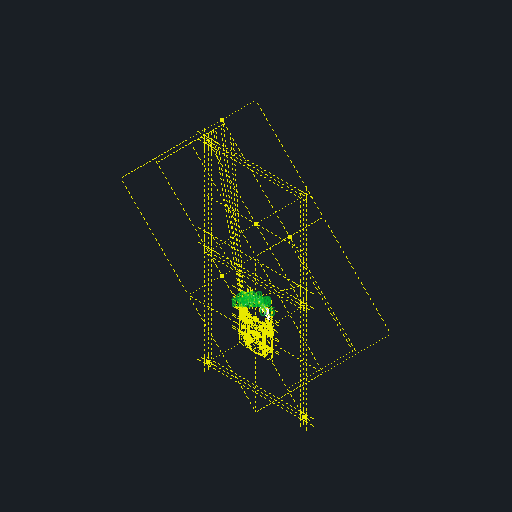
# Autodesk Inventor part: sensorcircuit
Saved by Autodesk Inventor 2023.5 (Build 275446000, 446)
## iProperties
Created: 2025-01-11
Part Number: sensorcircuit
Material: 一般
Document SubType Name: Modeling
Designer: IshiiLabHonda
Density: 1 g/cm^3
Appearance: 既定
Author: IshiiLabHonda
Autodesk Inventor part; units mm, degrees
ref_plane "YZ Plane" through (0, 0, 0) normal (1, 0, 0) x (0, 1, 0)
ref_plane "XZ Plane" through (0, 0, 0) normal (0, 1, 0) x (-1, 0, 0)
ref_plane "XY Plane" through (0, 0, 0) normal (0, 0, 1) x (1, 0, 0)
derived "circuit.ipt"
sketch "スケッチ1" plane through (0, 0, 0) normal (0, 0, 1) x (1, 0, 0)
  line L0 (0, 0) -> (0, 1) construction
  line L1 (0, 0) -> (1, 0) construction
  line L2 (-90, 90) -> (90, 90) construction
  line L3 (90, 90) -> (90, -90) construction
  line L4 (90, -90) -> (-90, -90) construction
  line L5 (-90, -90) -> (-90, 90) construction
  line L6 (-90, -90) -> (90, 90) construction
  line L7 (-90, 90) -> (90, -90) construction
  line L8 (-84, 96) -> (-84, 84) construction
  line L9 (-84, 84) -> (-96, 84) construction
  line L10 (-96, 84) -> (-96, 96) construction
  line L11 (-96, 96) -> (-84, 84) construction
  line L12 (-84, 96) -> (-96, 84) construction
  line L13 (-96, 96) -> (-84, 96) construction
  line L14 (-96, -96) -> (-96, -84) construction
  line L15 (-84, -96) -> (-96, -96) construction
  line L16 (-96, -96) -> (-84, -84) construction
  line L17 (-96, -84) -> (-84, -96) construction
  line L18 (-84, -84) -> (-84, -96) construction
  line L19 (-96, -84) -> (-84, -84) construction
  line L20 (96, -96) -> (84, -96) construction
  line L21 (96, -84) -> (96, -96) construction
  line L22 (96, -96) -> (84, -84) construction
  line L23 (84, -96) -> (96, -84) construction
  line L24 (84, -84) -> (96, -84) construction
  line L25 (84, -96) -> (84, -84) construction
  line L26 (96, 96) -> (96, 84) construction
  line L27 (84, 96) -> (96, 96) construction
  line L28 (96, 96) -> (84, 84) construction
  line L29 (96, 84) -> (84, 96) construction
  line L30 (84, 84) -> (84, 96) construction
  line L31 (96, 84) -> (84, 84) construction
  line L32 (-84, 84) -> (-84, -84) construction
  line L33 (-96, 84) -> (-96, -84) construction
  line L34 (-84, -84) -> (84, -84) construction
  line L35 (-84, -96) -> (84, -96) construction
  line L36 (96, 84) -> (96, -84) construction
  line L37 (84, 84) -> (84, -84) construction
  line L38 (-84, 96) -> (84, 96) construction
  line L39 (-84, 84) -> (84, 84) construction
  line L40 (-19, 15) -> (19, 15) construction
  line L41 (19, 15) -> (19, -15) construction
  line L42 (19, -15) -> (-19, -15) construction
  line L43 (-19, -15) -> (-19, 15) construction
  line L44 (-19, 15) -> (19, -15) construction
  line L45 (19, 15) -> (-19, -15) construction
  line L46 (-30.25, 11.5) -> (-19, 11.5) construction
  line L47 (-19, -11.5) -> (-30.25, -11.5) construction
  line L48 (-30.25, -11.5) -> (-30.25, 11.5) construction
  line L49 (-30.25, 11.5) -> (-19, -11.5) construction
  line L50 (-19, 11.5) -> (-30.25, -11.5) construction
  line L51 (30.25, 11.5) -> (19, 11.5) construction
  line L52 (19, -11.5) -> (30.25, -11.5) construction
  line L53 (30.25, -11.5) -> (30.25, 11.5) construction
  line L54 (30.25, 11.5) -> (19, -11.5) construction
  line L55 (19, 11.5) -> (30.25, -11.5) construction
  line L56 (-19, -10) -> (19, -10) construction
  line L57 (-19, -12.5) -> (19, -12.5) construction
  line L58 (-19, 10) -> (19, 10) construction
  line L59 (-19, 12.5) -> (19, 12.5) construction
  line L60 (-16.5, -15) -> (-16.5, 15) construction
  line L61 (16.5, -15) -> (16.5, 15) construction
  line L62 (-12.5, -10) -> (-12.5, -15) construction
  line L63 (-16.5, -10) -> (-12.5, -15) construction
  line L64 (-16.5, -15) -> (-12.5, -10) construction
  circle A0 centre (-14.5, -12.5) radius 0.8 construction
  line L65 (12.5, -10) -> (12.5, -15) construction
  line L66 (16.5, -10) -> (12.5, -15) construction
  line L67 (16.5, -15) -> (12.5, -10) construction
  circle A1 centre (14.5, -12.5) radius 0.8 construction
  line L68 (-12.5, 10) -> (-12.5, 15) construction
  line L69 (-16.5, 10) -> (-12.5, 15) construction
  line L70 (-16.5, 15) -> (-12.5, 10) construction
  circle A2 centre (-14.5, 12.5) radius 0.8 construction
  line L71 (12.5, 10) -> (12.5, 15) construction
  line L72 (16.5, 10) -> (12.5, 15) construction
  circle A3 centre (14.5, 12.5) radius 0.8 construction
  line L73 (16.5, 15) -> (12.5, 10) construction
  line L74 (-96, 276) -> (-84, 276) construction
  line L75 (-84, 276) -> (-84, 264) construction
  line L76 (-84, 264) -> (-96, 264) construction
  line L77 (-96, 264) -> (-96, 276) construction
  line L78 (-96, 276) -> (-84, 264) construction
  line L79 (-84, 276) -> (-96, 264) construction
  line L80 (-90, 90) -> (-90, 270) construction
  line L81 (-96, 264) -> (-96, 96) construction
  line L82 (-84, 264) -> (-84, 96) construction
  line L83 (96, 276) -> (84, 276) construction
  line L84 (84, 276) -> (84, 264) construction
  line L85 (84, 264) -> (96, 264) construction
  line L86 (96, 264) -> (96, 276) construction
  line L87 (96, 276) -> (84, 264) construction
  line L88 (84, 276) -> (96, 264) construction
  line L89 (90, 90) -> (90, 270) construction
  line L90 (96, 264) -> (96, 96) construction
  line L91 (84, 264) -> (84, 96) construction
  line L92 (-84, 276) -> (84, 276) construction
  line L93 (-84, 264) -> (84, 264) construction
  line L94 (-90, 270) -> (90, 270) construction
  line L95 (-90, 270) -> (90, 90) construction
  line L96 (-90, 90) -> (90, 270) construction
  circle A4 centre (0, 0) radius 15 construction
  line L97 (-96, 120) -> (96, 120) construction
  line L98 (0, 127.2792) -> (0, -127.2792) construction
  line L99 (-127.2792, 0) -> (127.2792, 0) construction
  line L100 (127.2792, 0) -> (0, -127.2792) construction
  line L101 (0, -127.2792) -> (-127.2792, 0) construction
  line L102 (-127.2792, 0) -> (0, 127.2792) construction
  line L103 (0, 127.2792) -> (127.2792, 0) construction
  line L104 (127.2792, 254.5584) -> (254.5584, 127.2792) construction
  line L105 (254.5584, 127.2792) -> (127.2792, 0) construction
  line L106 (127.2792, 0) -> (0, 127.2792) construction
  line L107 (0, 127.2792) -> (127.2792, 254.5584) construction
  line L108 (-127.2792, 254.5584) -> (0, 127.2792) construction
  line L109 (0, 127.2792) -> (-127.2792, 0) construction
  line L110 (-127.2792, 0) -> (-254.5584, 127.2792) construction
  line L111 (-254.5584, 127.2792) -> (-127.2792, 254.5584) construction
  line L112 (0, 381.8377) -> (127.2792, 254.5584) construction
  line L113 (127.2792, 254.5584) -> (0, 127.2792) construction
  line L114 (0, 127.2792) -> (-127.2792, 254.5584) construction
  line L115 (-127.2792, 254.5584) -> (0, 381.8377) construction
  line L116 (190.9188, 63.6396) -> (63.6396, 190.9188) construction
  line L117 (-190.9188, 190.9188) -> (-63.6396, 63.6396) construction
  line L118 (59.397, -59.397) -> (186.6762, 67.8823) construction
  line L119 (59.397, 186.6762) -> (186.6762, 59.397) construction
  line L120 (63.6396, 190.9188) -> (-63.6396, 318.1981) construction
  line L121 (-186.6762, 186.6762) -> (-59.397, 313.9554) construction
  point P0 (-90, -90)
  point P1 (90, -90)
  point P2 (-24.625, 0)
  point P3 (-84, 120)
  point P4 (84, 120)
  point P5 (0, 0)
sketch "スケッチ5" plane through (0, 0, 0) normal (0, 0, 1) x (1, 0, 0)
  line L0 (0, 0) -> (0, 1) construction
  line L1 (30.25, 11.5) -> (19, 11.5) construction
  line L2 (19, 11.5) -> (30.25, -11.5) construction
  line L3 (30.25, 11.5) -> (19, -11.5) construction
  line L4 (30.25, -11.5) -> (30.25, 11.5) construction
  line L5 (19, -11.5) -> (30.25, -11.5) construction
  line L6 (-90, 90) -> (90, 90) construction
  line L7 (-90, -90) -> (90, 90) construction
  line L8 (-90, 90) -> (90, -90) construction
  line L9 (-84, 84) -> (-84, -84) construction
  line L10 (-96, 84) -> (-96, -84) construction
  line L11 (-90, -90) -> (-90, 90) construction
  line L12 (-84, 84) -> (-96, 84) construction
  line L13 (-96, 84) -> (-96, 96) construction
  line L14 (84, 84) -> (84, -84) construction
  line L15 (90, 90) -> (90, -90) construction
  line L16 (96, 84) -> (84, 84) construction
  line L17 (96, 84) -> (96, -84) construction
  line L18 (90, -90) -> (-90, -90) construction
  line L19 (-84, -84) -> (84, -84) construction
  line L20 (-84, -96) -> (84, -96) construction
  line L21 (-84, -84) -> (-84, -96) construction
  line L22 (-96, -96) -> (-96, -84) construction
  line L23 (-84, -96) -> (-96, -96) construction
  line L24 (-96, -96) -> (-84, -84) construction
  line L25 (-96, -84) -> (-84, -96) construction
  line L26 (-96, -84) -> (-84, -84) construction
  line L27 (0, 0) -> (1, 0) construction
  line L28 (-84, 264) -> (-96, 264) construction
  line L29 (-96, 276) -> (-84, 276) construction
  line L30 (-96, 264) -> (-96, 276) construction
  line L31 (-84, 276) -> (-96, 264) construction
  line L32 (-96, 276) -> (-84, 264) construction
  line L33 (-84, 276) -> (-84, 264) construction
  line L34 (84, -96) -> (84, -84) construction
  line L35 (96, -96) -> (84, -96) construction
  line L36 (96, -84) -> (96, -96) construction
  line L37 (96, -96) -> (84, -84) construction
  line L38 (84, -96) -> (96, -84) construction
  line L39 (84, -84) -> (96, -84) construction
  line L40 (-19, 15) -> (19, 15) construction
  line L41 (19, 15) -> (19, -15) construction
  line L42 (16.5, 15) -> (12.5, 10) construction
  line L43 (12.5, 10) -> (12.5, 15) construction
  line L44 (16.5, 10) -> (12.5, 15) construction
  line L45 (16.5, -15) -> (16.5, 15) construction
  line L46 (-19, 10) -> (19, 10) construction
  line L47 (-19, 12.5) -> (19, 12.5) construction
  circle A0 centre (0, 0) radius 15 construction
  line L48 (-19, -10) -> (19, -10) construction
  line L49 (-19, -12.5) -> (19, -12.5) construction
  line L50 (19, -15) -> (-19, -15) construction
  line L51 (-19, 15) -> (19, -15) construction
  line L52 (19, 15) -> (-19, -15) construction
  line L53 (-16.5, -15) -> (-16.5, 15) construction
  line L54 (-19, -15) -> (-19, 15) construction
  line L55 (-30.25, 11.5) -> (-19, 11.5) construction
  line L56 (-19, -11.5) -> (-30.25, -11.5) construction
  line L57 (-30.25, -11.5) -> (-30.25, 11.5) construction
  line L58 (-30.25, 11.5) -> (-19, -11.5) construction
  line L59 (-19, 11.5) -> (-30.25, -11.5) construction
  line L60 (-12.5, 10) -> (-12.5, 15) construction
  circle A1 centre (-14.5, 12.5) radius 0.8 construction
  line L61 (-16.5, 10) -> (-12.5, 15) construction
  line L62 (-16.5, 15) -> (-12.5, 10) construction
  circle A2 centre (14.5, 12.5) radius 0.8 construction
  line L63 (-84, 96) -> (-96, 84) construction
  line L64 (-96, 96) -> (-84, 96) construction
  line L65 (-84, 96) -> (-84, 84) construction
  line L66 (-96, 96) -> (-84, 84) construction
  line L67 (-96, 264) -> (-96, 96) construction
  line L68 (-84, 264) -> (-84, 96) construction
  line L69 (-84, 96) -> (84, 96) construction
  line L70 (-84, 84) -> (84, 84) construction
  line L71 (84, 84) -> (84, 96) construction
  line L72 (96, 96) -> (96, 84) construction
  line L73 (96, 96) -> (84, 84) construction
  line L74 (96, 84) -> (84, 96) construction
  line L75 (-96, 120) -> (96, 120) construction
  line L76 (84, 96) -> (96, 96) construction
  line L77 (-84, 264) -> (84, 264) construction
  line L78 (84, 264) -> (84, 96) construction
  line L79 (-84, 276) -> (84, 276) construction
  line L80 (96, 264) -> (96, 96) construction
  line L81 (-90, 270) -> (90, 270) construction
  line L82 (-90, 270) -> (90, 90) construction
  line L83 (-90, 90) -> (90, 270) construction
  line L84 (90, 90) -> (90, 270) construction
  line L85 (-90, 90) -> (-90, 270) construction
  line L86 (84, 264) -> (96, 264) construction
  line L87 (96, 276) -> (84, 276) construction
  line L88 (96, 276) -> (84, 264) construction
  line L89 (84, 276) -> (96, 264) construction
  line L90 (96, 264) -> (96, 276) construction
  line L91 (84, 276) -> (84, 264) construction
  circle A3 centre (-14.5, -12.5) radius 0.8 construction
  line L92 (-12.5, -10) -> (-12.5, -15) construction
  line L93 (-16.5, -15) -> (-12.5, -10) construction
  line L94 (12.5, -10) -> (12.5, -15) construction
  circle A4 centre (14.5, -12.5) radius 0.8 construction
  line L95 (16.5, -15) -> (12.5, -10) construction
  line L96 (16.5, -10) -> (12.5, -15) construction
  line L97 (-16.5, -10) -> (-12.5, -15) construction
  line L98 (-12.9773, 53.9269) -> (-10.5199, 55.6476) construction
  line L99 (-8.7991, 53.1902) -> (-12.9773, 53.9269) construction
  circle A5 centre (-10.8882, 53.5585) radius 0.8 construction
  line L100 (-8.7991, 53.1902) -> (-11.2566, 51.4694) projected
  line L101 (-10.5199, 55.6476) -> (-11.2566, 51.4694) construction
  line L102 (-11.2566, 51.4694) -> (-12.9773, 53.9269) projected
  line L103 (-30.25, 44.8844) -> (-31, 44.3592) construction
  line L104 (-12.9471, 57) -> (-30.25, 44.8844) construction
  line L105 (-30.25, 57) -> (-31, 57) construction
  line L106 (-10.5199, 55.6476) -> (-8.7991, 53.1902) projected
  line L107 (-30.25, 57) -> (30.25, 57) construction
  line L108 (-6.2185, 52.5556) -> (-11.543, 48.8274) projected
  line L109 (-11.543, 48.8274) -> (-15.558, 54.5615) projected
  line L110 (-10.2335, 58.2897) -> (-6.2185, 52.5556) projected
  line L111 (1.0005, 57) -> (-30.25, 35.1182) construction
  line L112 (-1.0005, 57) -> (30.25, 35.1182) construction
  line L113 (-19, 15) -> (19, 15) construction
  line L114 (12.5, 10) -> (12.5, 15) construction
  line L115 (-19, 10) -> (19, 10) construction
  circle A6 centre (-14.5, 12.5) radius 0.8 construction
  line L116 (-12.5, 10) -> (-12.5, 15) construction
  line L117 (-16.5, 10) -> (-12.5, 15) construction
  line L118 (-16.5, 15) -> (-12.5, 10) construction
  line L119 (-19, 12.5) -> (19, 12.5) construction
  line L120 (30.25, 57) -> (31, 57) construction
  line L121 (30.25, 11.5) -> (30.25, 57) construction
  line L122 (-6.1403, 52) -> (6.1403, 52) construction
  line L123 (-30.25, 35.1182) -> (-31, 34.593) construction
  line L124 (-30.25, 11.5) -> (-30.25, 57) construction
  line L125 (-6.7921, 53.3748) -> (-12.1165, 49.6465) construction
  line L126 (-10.8882, 53.5585) -> (-10.4294, 52.9032) construction
  line L127 (-10.8882, 53.5585) -> (-10.2329, 54.0174) construction
  line L128 (-6.2185, 52.5556) -> (-15.558, 54.5615) construction
  line L129 (-9.6599, 57.4705) -> (-14.9844, 53.7423) construction
  line L130 (-15.558, 54.5615) -> (-10.2335, 58.2897) construction
  line L131 (-10.2335, 58.2897) -> (-11.543, 48.8274) construction
  line L132 (-30.25, 11.5) -> (-19, 11.5) construction
  line L133 (-30.25, 11.5) -> (-19, -11.5) construction
  line L134 (30.25, 11.5) -> (19, 11.5) construction
  line L135 (30.25, -11.5) -> (30.25, 11.5) construction
  line L136 (19, 11.5) -> (30.25, -11.5) construction
  line L137 (30.25, 11.5) -> (19, -11.5) construction
  line L138 (0, 0) -> (0, 1) construction
  line L139 (0, 0) -> (1, 0) construction
  circle A7 centre (0, 0) radius 7.5 construction
  circle A8 centre (0, 0) radius 15 construction
  line L140 (-16.5, -15) -> (-16.5, 15) construction
  circle A9 centre (14.5, 12.5) radius 0.8 construction
  line L141 (-12.5, -10) -> (-12.5, -15) construction
  line L142 (12.5, -10) -> (12.5, -15) construction
  line L143 (16.5, 10) -> (12.5, 15) construction
  line L144 (-16.5, -15) -> (-12.5, -10) construction
  line L145 (16.5, -10) -> (12.5, -15) construction
  line L146 (16.5, 15) -> (12.5, 10) construction
  line L147 (-19, -12.5) -> (19, -12.5) construction
  line L148 (19, -15) -> (-19, -15) construction
  line L149 (-19, 11.5) -> (-30.25, -11.5) construction
  line L150 (19, -11.5) -> (30.25, -11.5) construction
  line L151 (-19, -11.5) -> (-30.25, -11.5) construction
  line L152 (-30.25, -11.5) -> (-30.25, 11.5) construction
  line L153 (16.5, -15) -> (16.5, 15) construction
  line L154 (19, 15) -> (19, -15) construction
  line L155 (-19, -15) -> (-19, 15) construction
  line L156 (-19, 15) -> (19, -15) construction
  line L157 (19, 15) -> (-19, -15) construction
  line L158 (-31, -8.5) -> (31, -8.5) construction
  line L159 (-31, 8.5) -> (31, 8.5) construction
  line L160 (-31, -30) -> (31, -30) construction
  line L161 (-31, 57) -> (-31, -30) construction
  line L162 (31, 57) -> (31, -30) construction
  line L163 (84, -84) -> (96, -84) construction
  line L164 (84, -96) -> (96, -84) construction
  line L165 (96, -96) -> (84, -84) construction
  line L166 (96, -84) -> (96, -96) construction
  line L167 (96, -96) -> (84, -96) construction
  line L168 (-96, 84) -> (-96, -84) construction
  line L169 (-84, 84) -> (-84, -84) construction
  line L170 (-90, -90) -> (-90, 90) construction
  line L171 (-84, -84) -> (84, -84) construction
  line L172 (-84, -96) -> (84, -96) construction
  line L173 (-90, -90) -> (90, 90) construction
  line L174 (90, -90) -> (-90, -90) construction
  line L175 (-90, 90) -> (90, -90) construction
  line L176 (84, 84) -> (84, -84) construction
  line L177 (90, 90) -> (90, -90) construction
  line L178 (96, 84) -> (96, -84) construction
  line L179 (84, -96) -> (84, -84) construction
  line L180 (-19, -10) -> (19, -10) construction
  circle A10 centre (14.5, -12.5) radius 0.8 construction
  line L181 (16.5, -15) -> (12.5, -10) construction
  line L182 (-16.5, -10) -> (-12.5, -15) construction
  line L183 (-84, -84) -> (-84, -96) construction
  line L184 (-96, -84) -> (-84, -84) construction
  line L185 (-84, -96) -> (-96, -96) construction
  line L186 (-96, -96) -> (-84, -84) construction
  line L187 (-96, -84) -> (-84, -96) construction
  line L188 (-96, -96) -> (-96, -84) construction
  circle A11 centre (-14.5, -12.5) radius 0.8 construction
  line L189 (-96, 96) -> (-84, 96) construction
  line L190 (-84, 96) -> (-84, 84) construction
  line L191 (-84, 96) -> (-96, 84) construction
  line L192 (-96, 96) -> (-84, 84) construction
  line L193 (84, 96) -> (96, 96) construction
  line L194 (96, 84) -> (84, 84) construction
  line L195 (96, 96) -> (96, 84) construction
  line L196 (96, 96) -> (84, 84) construction
  line L197 (96, 84) -> (84, 96) construction
  line L198 (-96, 120) -> (96, 120) construction
  line L199 (-84, 96) -> (84, 96) construction
  line L200 (-90, 90) -> (90, 90) construction
  line L201 (-84, 84) -> (-96, 84) construction
  line L202 (-96, 84) -> (-96, 96) construction
  line L203 (-84, 84) -> (84, 84) construction
  line L204 (84, 120) -> (-30.25, 40.0013) construction
  line L205 (-84, 120) -> (30.25, 40.0013) construction
  line L206 (84, 84) -> (84, 96) construction
  line L207 (-84, 264) -> (-96, 264) construction
  line L208 (-90, 90) -> (-90, 270) construction
  line L209 (-96, 264) -> (-96, 96) construction
  line L210 (-84, 264) -> (-84, 96) construction
  line L211 (96, 264) -> (96, 96) construction
  line L212 (84, 264) -> (84, 96) construction
  line L213 (90, 90) -> (90, 270) construction
  line L214 (-90, 90) -> (90, 270) construction
  line L215 (-90, 270) -> (90, 90) construction
  line L216 (-84, 264) -> (84, 264) construction
  line L217 (-90, 270) -> (90, 270) construction
  line L218 (-96, 264) -> (-96, 276) construction
  line L219 (-96, 276) -> (-84, 276) construction
  line L220 (-96, 276) -> (-84, 264) construction
  line L221 (-84, 276) -> (-96, 264) construction
  line L222 (-84, 276) -> (-84, 264) construction
  line L223 (-84, 276) -> (84, 276) construction
  line L224 (84, 264) -> (96, 264) construction
  line L225 (96, 264) -> (96, 276) construction
  line L226 (96, 276) -> (84, 264) construction
  line L227 (96, 276) -> (84, 276) construction
  line L228 (84, 276) -> (96, 264) construction
  line L229 (84, 276) -> (84, 264) construction
  line L230 (-31, 8.5) -> (-19, 8.5) construction
  line L231 (-31, -8.5) -> (-19, -8.5) construction
  line L232 (-19, 8.5) -> (-19, -8.5) construction
  circle A12 centre (0, 0) radius 7.5 construction
  line L233 (31, 8.5) -> (19, 8.5) construction
  line L234 (31, -8.5) -> (19, -8.5) construction
  line L235 (19, 8.5) -> (19, -8.5) construction
  line L236 (31, 8.5) -> (31, 8.5) projected
  line L237 (-31, -8.5) -> (-12.9594, -30) construction
  line L238 (-12.9594, -30) -> (12.9594, -30) construction
  line L239 (31, -8.5) -> (12.9594, -30) construction
  circle A13 centre (-14.5, 12.5) radius 1 construction
  circle A14 centre (14.5, 12.5) radius 1 construction
  circle A15 centre (-14.5, -12.5) radius 1 construction
  circle A16 centre (14.5, -12.5) radius 1 construction
  line L240 (-10.5199, 55.6476) -> (-12.9773, 53.9269) projected
  line L241 (-12.9773, 53.9269) -> (-11.2566, 51.4694) construction
  line L242 (-11.2566, 51.4694) -> (-8.7991, 53.1902) construction
  line L243 (-8.7991, 53.1902) -> (-10.5199, 55.6476) construction
  line L244 (-26.25, 26.5) -> (-26.3613, 27.2922) construction
  line L245 (-26.25, 26.5) -> (-25.4578, 26.6113) construction
  circle A17 centre (-26.25, 26.5) radius 0.8 construction
  line L246 (-24.1223, 29.3236) -> (-23.4264, 24.3723) construction
  line L247 (-28.3777, 23.6764) -> (-29.0736, 28.6277) construction
  line L248 (-24.1223, 29.3236) -> (-28.3777, 23.6764) construction
  line L249 (-29.0736, 28.6277) -> (-24.1223, 29.3236) construction
  line L250 (-23.4264, 24.3723) -> (-28.3777, 23.6764) construction
  line L251 (-29.0736, 28.6277) -> (-23.4264, 24.3723) construction
  line L252 (10.5199, 55.6476) -> (12.9773, 53.9269) projected
  line L253 (12.9773, 53.9269) -> (11.2566, 51.4694) projected
  line L254 (11.2566, 51.4694) -> (8.7991, 53.1902) projected
  line L255 (8.7991, 53.1902) -> (10.5199, 55.6476) projected
  line L256 (-29.0736, 28.6277) -> (-28.3777, 23.6764) construction
  line L257 (-24.1223, 29.3236) -> (-19.1709, 30.0195) construction
  line L258 (-19.1709, 30.0195) -> (-18.4751, 25.0681) construction
  line L259 (-18.4751, 25.0681) -> (-23.4264, 24.3723) construction
  line L260 (28.3777, 23.6764) -> (23.4264, 24.3723) construction
  line L261 (18.4751, 25.0681) -> (23.4264, 24.3723) construction
  line L262 (19.1709, 30.0195) -> (18.4751, 25.0681) construction
  line L263 (24.1223, 29.3236) -> (19.1709, 30.0195) construction
  line L264 (24.1223, 29.3236) -> (29.0736, 28.6277) construction
  line L265 (29.0736, 28.6277) -> (28.3777, 23.6764) construction
  line L266 (-29.0736, 28.6277) -> (-19.1709, 30.0195) construction
  line L267 (-18.4751, 25.0681) -> (-19.1709, 30.0195) projected
  line L268 (-18.4751, 25.0681) -> (-28.3777, 23.6764) construction
  line L269 (19.1709, 30.0195) -> (29.0736, 28.6277) construction
  line L270 (28.3777, 23.6764) -> (29.0736, 28.6277) construction
  line L271 (28.3777, 23.6764) -> (18.4751, 25.0681) construction
  line L272 (19.1709, 30.0195) -> (18.4751, 25.0681) construction
  line L273 (-9.6771, 59.2897) -> (9.6771, 59.2897) construction
  line L274 (-9.6771, 59.2897) -> (-9.6771, 59.2897) construction
  line L275 (-3.6771, 59.2897) -> (-0.9296, 58.2897) construction
  line L276 (-0.9296, 58.2897) -> (0.9296, 58.2897) construction
  line L277 (0.9296, 58.2897) -> (3.6771, 59.2897) construction
  line L278 (-4.6137, 54.2897) -> (4.6137, 54.2897) construction
  line L279 (-18.1736, 44.795) -> (-4.6137, 54.2897) construction
  line L280 (-31, 8.5) -> (-22.0451, 50.6295) construction
  line L281 (-22.0451, 50.6295) -> (-9.6771, 59.2897) construction
  line L282 (31, 8.5) -> (22.0451, 50.6295) construction
  line L283 (-18.1736, 44.795) -> (-23.6565, 19) construction
  line L284 (18.1736, 44.795) -> (23.6565, 19) construction
  line L285 (-23.6565, 19) -> (23.6565, 19) construction
  line L286 (-17.5234, -20) -> (17.5234, -20) construction
  line L287 (17.5234, -20) -> (12.3689, -25) construction
  line L288 (12.3689, -25) -> (-12.3689, -25) construction
  line L289 (-12.3689, -25) -> (-17.5234, -20) construction
  line L290 (-31, -8.5) -> (-31, -12.5) construction
  line L291 (-31, -12.5) -> (-12.9594, -30) construction
  line L292 (31, -8.5) -> (31, -12.5) construction
  line L293 (31, -12.5) -> (12.9594, -30) construction
  line L294 (-31, 8.5) -> (-31, 26.5) construction
  line L295 (-31, 26.5) -> (-26.3435, 30.4073) construction
  line L296 (31, 8.5) -> (31, 26.5) construction
  line L297 (31, 26.5) -> (26.3435, 30.4073) construction
  line L298 (-8.9594, -30) -> (-7.4594, -28.5) construction
  line L299 (-7.4594, -28.5) -> (7.4594, -28.5) construction
  line L300 (7.4594, -28.5) -> (8.9594, -30) construction
  line L301 (18.1736, 44.795) -> (4.6137, 54.2897) construction
  line L302 (22.0451, 50.6295) -> (9.6771, 59.2897) construction
  line L303 (-23.6565, 19) -> (-24.8255, 13.5) construction
  line L304 (-24.8255, 13.5) -> (-20.8255, 13.5) construction
  line L305 (-20.8255, 13.5) -> (-15.3255, 19) construction
  line L306 (23.6565, 19) -> (24.8255, 13.5) construction
  line L307 (24.8255, 13.5) -> (20.8255, 13.5) construction
  line L308 (20.8255, 13.5) -> (15.3255, 19) construction
  line L309 (-17.5234, -20) -> (-24.2242, -13.5) construction
  line L310 (-24.2242, -13.5) -> (-21.2242, -13.5) construction
  line L311 (-21.2242, -13.5) -> (-11.5234, -20) construction
  line L312 (17.5234, -20) -> (24.2242, -13.5) construction
  line L313 (24.2242, -13.5) -> (21.2242, -13.5) construction
  line L314 (21.2242, -13.5) -> (11.5234, -20) construction
  line L315 (-10.5173, 23.5) -> (-4.5173, 23.5) projected
  line L316 (-4.5173, 23.5) -> (-2, 26.5) projected
  line L317 (-2, 26.5) -> (2, 26.5) projected
  line L318 (2, 26.5) -> (4.5173, 23.5) projected
  line L319 (4.5173, 23.5) -> (10.5173, 23.5) projected
  line L320 (0, 0) -> (1, 0) construction
  line L321 (0, 0) -> (0, 1) construction
  line L322 (-30.5, 13) -> (-20, 13) projected
  line L323 (-20, 13) -> (-20, 17.5) projected
  line L324 (-20, 17.5) -> (-16, 17.5) projected
  line L325 (20, 17.5) -> (16, 17.5) projected
  line L326 (20, 13) -> (20, 17.5) projected
  line L327 (30.5, 13) -> (20, 13) projected
  circle A18 centre (0, 0) radius 1.5 projected
  line L328 (-16, 17.5) -> (-16, -17) projected
  line L329 (16, 17.5) -> (16, -17) projected
  line L330 (-30.5, 20.6916) -> (-10.5173, 23.5) projected
  line L331 (30.5, 20.6916) -> (10.5173, 23.5) projected
  circle A19 centre (-10.0234, -17) radius 0.475 construction
  circle A20 centre (-10.0234, -17) radius 0.8 projected
  circle A21 centre (-10.0234, -17) radius 1.5 projected
  line L332 (-11.5234, -20) -> (-11.5234, -15) construction
  circle A22 centre (10.0234, -17) radius 0.475 construction
  circle A23 centre (10.0234, -17) radius 0.8 projected
  circle A24 centre (10.0234, -17) radius 1.5 projected
  circle A25 centre (-9, 15.5) radius 0.475 construction
  circle A26 centre (-9, 15.5) radius 0.8 projected
  circle A27 centre (-9, 15.5) radius 1.5 projected
  circle A28 centre (9, 15.5) radius 0.475 construction
  circle A29 centre (9, 15.5) radius 0.8 projected
  circle A30 centre (9, 15.5) radius 1.5 projected
  line L333 (-9.091, 59.0897) -> (-21.597, 50.3329)
  line L334 (-21.597, 50.3329) -> (-23.6677, 40.5908)
  line L335 (-3.4267, 53.2897) -> (3.4267, 53.2897)
  line L336 (23.5225, 41.2738) -> (21.597, 50.3329)
  line L337 (21.597, 50.3329) -> (9.091, 59.0897)
  line L338 (9.091, 59.0897) -> (-9.091, 59.0897)
  circle A31 centre (-17.3746, 49.0168) radius 0.475 construction
  circle A32 centre (-17.3746, 49.0168) radius 0.8 projected
  circle A33 centre (-17.3746, 49.0168) radius 1.5 construction
  circle A34 centre (17.3746, 49.0168) radius 0.475 construction
  circle A35 centre (17.3746, 49.0168) radius 0.8 projected
  circle A36 centre (17.3746, 49.0168) radius 1.5 construction
  line L339 (-11.6471, 47.5337) -> (-10.6006, 47.0457)
  line L340 (-10.6006, 47.0457) -> (-4.8665, 51.0607)
  line L341 (-4.8665, 51.0607) -> (-4.9672, 52.211)
  line L342 (-16.3711, 44.2259) -> (-11.6471, 47.5337)
  line L343 (-4.9672, 52.211) -> (-3.4267, 53.2897)
  line L344 (11.6471, 47.5337) -> (10.6006, 47.0457)
  line L345 (10.6006, 47.0457) -> (4.8665, 51.0607)
  line L346 (4.8665, 51.0607) -> (4.9672, 52.211)
  line L347 (4.9672, 52.211) -> (3.4267, 53.2897)
  line L348 (0, 59.0897) -> (-10.3891, 58.1808)
  line L349 (0, 59.0897) -> (10.3891, 58.1808)
  line L350 (-10.3891, 58.1808) -> (-2.3891, 58.1808)
  line L351 (-2.3891, 58.1808) -> (0, 59.0897)
  line L352 (10.3891, 58.1808) -> (2.3891, 58.1808)
  line L353 (2.3891, 58.1808) -> (0, 59.0897)
  line L354 (-3.1638, 53.2897) -> (-1, 51.4741)
  line L355 (-1, 51.4741) -> (1, 51.4741)
  line L356 (1, 51.4741) -> (3.1638, 53.2897)
  line L357 (-10, -29) -> (10, -29) projected
  line L358 (-16, -17) -> (-22.863, -17) projected
  line L359 (-22.863, -17) -> (-22.863, -19) projected
  line L360 (16, -17) -> (22.863, -17) projected
  line L361 (22.863, -17) -> (22.863, -19) projected
  line L362 (-12.8008, -25) -> (-18.1572, -23.5648) projected
  line L363 (-18.1572, -23.5648) -> (-22.863, -19) projected
  line L364 (12.8008, -25) -> (18.1572, -23.5648) projected
  line L365 (18.1572, -23.5648) -> (22.863, -19) projected
  line L366 (-30.5, 13) -> (-30.5, 20.6916) projected
  line L367 (30.5, 13) -> (30.5, 20.6916) projected
  line L368 (-16.3711, 44.2259) -> (-16.2403, 42.7317)
  line L369 (-16.2403, 42.7317) -> (-24.4318, 36.9959)
  line L370 (-24.4318, 36.9959) -> (-23.6677, 40.5908)
  line L371 (16.3711, 44.2259) -> (16.2403, 42.7317)
  line L372 (16.2403, 42.7317) -> (24.4318, 36.9959)
  line L373 (11.6471, 47.5337) -> (16.3711, 44.2259)
  line L374 (23.5225, 41.2738) -> (24.4318, 36.9959)
  line L375 (-12.8008, -25) -> (-10, -29) projected
  line L376 (10, -29) -> (12.8008, -25) projected
  line L377 (-1.25, 25) -> (1.25, 25) projected
  line L378 (2, 24.25) -> (2, 24.25) projected
  line L379 (1.25, 23.5) -> (-1.25, 23.5) projected
  line L380 (-2, 24.25) -> (-2, 24.25) projected
  arc A37 (-1.25, 25) -> (-2, 24.25) centre (-1.25, 24.25) ccw projected
  arc A38 (-2, 24.25) -> (-1.25, 23.5) centre (-1.25, 24.25) ccw projected
  arc A39 (1.25, 23.5) -> (2, 24.25) centre (1.25, 24.25) ccw projected
  arc A40 (2, 24.25) -> (1.25, 25) centre (1.25, 24.25) ccw projected
  line L381 (-30.5, 20.6916) -> (-28.3474, 27.0531) projected
  line L382 (-28.3474, 27.0531) -> (-19.435, 28.3057) projected
  line L383 (-19.435, 28.3057) -> (-15.6123, 22.7839) projected
  line L384 (30.5, 20.6916) -> (28.3474, 27.0531) projected
  line L385 (28.3474, 27.0531) -> (19.435, 28.3057) projected
  line L386 (19.435, 28.3057) -> (15.6123, 22.7839) projected
  line L387 (-30.8721, 30.6471) -> (-17.9987, 32.4563) projected
  line L388 (-17.9987, 32.4563) -> (-16.6765, 23.0488) projected
  line L389 (-16.6765, 23.0488) -> (-29.55, 21.2395) projected
  line L390 (-29.55, 21.2395) -> (-30.8721, 30.6471) projected
  line L391 (-22.0451, 50.6295) -> (-18.1736, 44.795) construction
  line L392 (-21.8107, 27.6837) -> (-26, 24.1685) construction
  line L393 (-26, 24.1685) -> (-26, 13.5) construction
  line L394 (-24.8255, 13.5) -> (-26, 13.5) construction
  line L395 (21.8107, 27.6837) -> (26, 24.1685) projected
  line L396 (26, 24.1685) -> (26, 13.5) projected
  line L397 (24.8255, 13.5) -> (26, 13.5) projected
  circle A41 centre (-28.5, 18.5) radius 0.475 construction
  circle A42 centre (-28.5, 18.5) radius 0.8 projected
  circle A43 centre (-28.5, 18.5) radius 1.5 projected
  line L398 (-19.435, 28.3057) -> (-10.5173, 23.5) projected
  line L399 (19.435, 28.3057) -> (10.5173, 23.5) projected
  circle A44 centre (28.5, 18.5) radius 0.8 projected
  circle A45 centre (28.5, 18.5) radius 1.5 projected
  circle A46 centre (28.5, 18.5) radius 0.475 construction
  line L400 (-12.9471, 57) -> (12.9471, 57) projected
  line L401 (10.2335, 58.2897) -> (6.2185, 52.5556) projected
  line L402 (6.2185, 52.5556) -> (11.543, 48.8274) projected
  line L403 (11.543, 48.8274) -> (15.558, 54.5615) projected
  circle A47 centre (-6.875, 0) radius 0.9 projected
  circle A48 centre (-6.875, 0) radius 0.8 construction
  circle A49 centre (6.875, 0) radius 0.8 construction
  circle A50 centre (6.875, 0) radius 0.9 projected
  circle A51 centre (0, 0) radius 5.75 projected
  circle A52 centre (-6.875, 0) radius 0.625 construction
  circle A53 centre (0, 0) radius 4.25 projected
  line L404 (30.8721, 30.6471) -> (17.9987, 32.4563) projected
  line L405 (17.9987, 32.4563) -> (16.6765, 23.0488) projected
  line L406 (16.6765, 23.0488) -> (29.55, 21.2395) projected
  line L407 (29.55, 21.2395) -> (30.8721, 30.6471) projected
  point P0 (-90, -90)
  point P1 (90, -90)
  point P2 (-24.625, 0)
  point P3 (-8.226, 55.4227)
  point P4 (-5.9733, 57)
  point P5 (0, 61.1826)
  point P6 (-24.625, 0)
  point P7 (-90, -90)
  point P8 (90, -90)
  point P9 (-5.9733, 57)
  point P10 (5.9733, 57)
  point P11 (10.3891, 58.1808)
  point P12 (10.3891, 58.1808)
  point P13 (-2, 25)
  point P14 (-2, 23.5)
  point P15 (0.6109, 58.1808)
  point P16 (-0.6109, 58.1808)
  point P17 (0.6109, 58.1808)
  point P18 (10.1572, 58.1808)
  point P19 (-10.1572, 58.1808)
  dimension "d2" = 0.5
  dimension "d3" = 0.5
  dimension "d5" = 0.5
  dimension "d13" = 1
  dimension "d14" = 0.5
  dimension "d15" = 120
  dimension "d16" = 120
  dimension "d17" = 0.5
  dimension "d18" = 1.5
  dimension "d19" = 7
  dimension "d21" = 0.2
  dimension "d22" = 5
  dimension "d26" = 8
  dimension "d29" = 40
  dimension "d34" = 2
  dimension "d35" = 6.3276
  dimension "d39" = 120
  dimension "d40" = 10
  dimension "d41" = 1.5
  constraints: 62 end point, 13 horizontal alignment, 11 parallel, 3 point on line, 1 coincident, 1 collinear, 1 horizontal, 1 midpoint, 1 symmetric about line, 34 other
  measures "d2" distance between parallel lines of L333 L104
  measures "d3" distance between parallel lines of L280 L334
  measures "d5" distance between parallel lines of L282 L336
  measures "d13" distance between parallel lines of L335 L278
  measures "d14" distance between parallel lines of L343 L111
  measures "d15" angle of L341 L343
  measures "d16" angle of L342 L339
  measures "d17" distance between parallel lines of L342 L111
  measures "d18" distance between parallel lines of L340 L111
  measures "d19" distance of L339.end L340.end
  measures "d21" distance between parallel lines of L338 L273
  measures "d22" angle of L348 L338
  measures "d26" distance of L348.end L350.end
  measures "d29" angle of L354 L335
  measures "d34" distance of L354.end L355.end
  measures "d35" distance of L356.end L354.start
  measures "d39" angle of L368 L342
  measures "d40" distance of L368.end L369.end
  measures "d41" distance of L342.start L368.end
extrude "押し出し4" add sketch "スケッチ5" against normal blind 0.6 contours L110 L400 L401 L402 L403 L337 L336 L374 L372 L371 L373 L344 L345 L346 L347 L335 L343 L341 L340 L339 L342 L368 L369 L370 L334 L333 L109 L108 | L108 L109 L333 L400 L110 | L400 L333 L350 L110 | L110 L350 L351 L353 L352 L401 L400 | L350 L348 L110 | L110 L348 L351 L350 | L401 L352 L337 L400 | L400 L337 L403 L402 L401 | L348 L333 L110 | L110 L333 L338 L348 | L401 L349 L352 | L352 L353 L349 L401 | L338 L337 L401 L349 | L349 L401 L337
extrude "押し出し5" cut sketch "スケッチ5" against normal blind 0.6 contours L350 L348 L110 | L110 L348 L351 L350 | L401 L349 L352 | L352 L353 L349 L401
extrude "押し出し6" add sketch "スケッチ5" against normal blind 0.6 contours L335 L356 L355 L354
extrude "押し出し8" cut sketch "スケッチ5" against normal blind 0.6 contours L348 L333 L110 | L110 L333 L338 L348 | L338 L337 L401 L349 | L349 L401 L337
extrude "押し出し9" add sketch "スケッチ5" against normal blind 0.6 contours L350 L348 L110 | L110 L348 L351 L350 | L401 L349 L352 | L352 L353 L349 L401
extrude "押し出し10" cut sketch "スケッチ5" against normal blind 0.6 contours L350 L348 L110 | L110 L348 L351 L350 | L401 L349 L352 | L352 L353 L349 L401
extrude "押し出し11" cut sketch "スケッチ5" against normal blind 0.1 contours L401 L352 L337 L400 | L400 L337 L403 L402 L401
extrude "押し出し12" cut sketch "スケッチ5" against normal blind 0.1 contours L108 L109 L333 L400 L110 | L400 L333 L350 L110
sketch "スケッチ4" plane through (0, 0, 0) normal (0, 0, 1) x (1, 0, 0)
  line L0 (-84, 264) -> (-96, 264) construction
  line L1 (-90, 90) -> (-90, 270) construction
  line L2 (-96, 264) -> (-96, 96) construction
  line L3 (-96, 96) -> (-84, 96) construction
  line L4 (-84, 96) -> (-84, 84) construction
  line L5 (-84, 96) -> (-96, 84) construction
  line L6 (-96, 96) -> (-84, 84) construction
  line L7 (-84, 264) -> (-84, 96) construction
  line L8 (-84, 84) -> (-96, 84) construction
  line L9 (84, -84) -> (96, -84) construction
  line L10 (84, -96) -> (96, -84) construction
  line L11 (96, -96) -> (84, -84) construction
  line L12 (96, -84) -> (96, -96) construction
  line L13 (96, -96) -> (84, -96) construction
  line L14 (0, 0) -> (0, 1) construction
  line L15 (0, 0) -> (1, 0) construction
  line L16 (16.5, 15) -> (12.5, 10) construction
  line L17 (-96, 84) -> (-96, -84) construction
  line L18 (-84, 84) -> (-84, -84) construction
  line L19 (-90, -90) -> (-90, 90) construction
  line L20 (-90, 90) -> (90, 90) construction
  line L21 (-84, -84) -> (84, -84) construction
  line L22 (-84, -96) -> (84, -96) construction
  line L23 (-90, -90) -> (90, 90) construction
  line L24 (90, -90) -> (-90, -90) construction
  line L25 (-90, 90) -> (90, -90) construction
  line L26 (84, 84) -> (84, -84) construction
  line L27 (90, 90) -> (90, -90) construction
  line L28 (96, 84) -> (96, -84) construction
  line L29 (-96, 84) -> (-96, 96) construction
  line L30 (-84, -84) -> (-84, -96) construction
  line L31 (-96, -84) -> (-84, -84) construction
  line L32 (-84, -96) -> (-96, -96) construction
  line L33 (-96, -96) -> (-84, -84) construction
  line L34 (-96, -84) -> (-84, -96) construction
  line L35 (-96, -96) -> (-96, -84) construction
  line L36 (84, -96) -> (84, -84) construction
  line L37 (-19, -15) -> (-19, 15) construction
  line L38 (-30.25, 11.5) -> (-19, 11.5) construction
  line L39 (-19, -11.5) -> (-30.25, -11.5) construction
  line L40 (-19, 11.5) -> (-30.25, -11.5) construction
  line L41 (-30.25, 11.5) -> (-19, -11.5) construction
  line L42 (-30.25, -11.5) -> (-30.25, 11.5) construction
  line L43 (12.5, 10) -> (12.5, 15) construction
  circle A0 centre (14.5, 12.5) radius 0.8 construction
  line L44 (30.25, 11.5) -> (19, 11.5) construction
  line L45 (16.5, 10) -> (12.5, 15) construction
  circle A1 centre (14.5, -12.5) radius 0.8 construction
  line L46 (16.5, -15) -> (12.5, -10) construction
  line L47 (16.5, -10) -> (12.5, -15) construction
  line L48 (12.5, -10) -> (12.5, -15) construction
  circle A2 centre (-14.5, -12.5) radius 0.8 construction
  line L49 (-12.5, -10) -> (-12.5, -15) construction
  line L50 (-16.5, -15) -> (-12.5, -10) construction
  line L51 (-16.5, -10) -> (-12.5, -15) construction
  line L52 (96, 84) -> (84, 84) construction
  line L53 (96, 96) -> (96, 84) construction
  line L54 (84, 96) -> (96, 96) construction
  line L55 (96, 96) -> (84, 84) construction
  line L56 (84, 84) -> (84, 96) construction
  line L57 (96, 84) -> (84, 96) construction
  line L58 (-96, 264) -> (-96, 276) construction
  line L59 (-84, 276) -> (-84, 264) construction
  line L60 (-96, 276) -> (-84, 276) construction
  line L61 (-96, 276) -> (-84, 264) construction
  line L62 (-84, 276) -> (-96, 264) construction
  line L63 (-84, 84) -> (84, 84) construction
  line L64 (-84, 96) -> (84, 96) construction
  line L65 (84, 264) -> (84, 96) construction
  line L66 (90, 90) -> (90, 270) construction
  line L67 (-90, 90) -> (90, 270) construction
  line L68 (-90, 270) -> (90, 90) construction
  line L69 (96, 264) -> (96, 96) construction
  line L70 (-96, 120) -> (96, 120) construction
  line L71 (-84, 264) -> (84, 264) construction
  line L72 (-84, 276) -> (84, 276) construction
  line L73 (-90, 270) -> (90, 270) construction
  line L74 (84, 276) -> (84, 264) construction
  line L75 (84, 264) -> (96, 264) construction
  line L76 (96, 264) -> (96, 276) construction
  line L77 (96, 276) -> (84, 264) construction
  line L78 (96, 276) -> (84, 276) construction
  line L79 (84, 276) -> (96, 264) construction
  line L80 (-19, 15) -> (19, 15) construction
  line L81 (19, 15) -> (19, -15) construction
  line L82 (19, -15) -> (-19, -15) construction
  circle A3 centre (-14.5, 12.5) radius 0.8 construction
  line L83 (-16.5, 10) -> (-12.5, 15) construction
  line L84 (-12.5, 10) -> (-12.5, 15) construction
  line L85 (-16.5, 15) -> (-12.5, 10) construction
  circle A4 centre (0, 0) radius 15 construction
  line L86 (-19, 10) -> (19, 10) construction
  line L87 (-19, 12.5) -> (19, 12.5) construction
  line L88 (-19, 15) -> (19, -15) construction
  line L89 (19, 15) -> (-19, -15) construction
  line L90 (-19, -10) -> (19, -10) construction
  line L91 (-19, -12.5) -> (19, -12.5) construction
  line L92 (16.5, -15) -> (16.5, 15) construction
  line L93 (19, 11.5) -> (30.25, -11.5) construction
  line L94 (19, -11.5) -> (30.25, -11.5) construction
  line L95 (30.25, -11.5) -> (30.25, 11.5) construction
  line L96 (30.25, 11.5) -> (19, -11.5) construction
  line L97 (-16.5, -15) -> (-16.5, 15) construction
  line L98 (-84, 120) -> (30.25, 40.0013) construction
  line L99 (84, 120) -> (-30.25, 40.0013) construction
  line L100 (-30.25, 57) -> (30.25, 57) construction
  line L101 (1.0005, 57) -> (-30.25, 35.1182) construction
  line L102 (-1.0005, 57) -> (30.25, 35.1182) construction
  line L103 (-12.9471, 57) -> (-30.25, 44.8844) construction
  line L104 (-10.2335, 58.2897) -> (-6.2185, 52.5556) construction
  line L105 (-6.2185, 52.5556) -> (-11.543, 48.8274) construction
  line L106 (-11.543, 48.8274) -> (-15.558, 54.5615) construction
  line L107 (-15.558, 54.5615) -> (-10.2335, 58.2897) construction
  line L108 (-10.2335, 58.2897) -> (-11.543, 48.8274) construction
  line L109 (-6.2185, 52.5556) -> (-15.558, 54.5615) construction
  line L110 (-9.6599, 57.4705) -> (-14.9844, 53.7423) construction
  line L111 (-6.7921, 53.3748) -> (-12.1165, 49.6465) construction
  line L112 (-10.8882, 53.5585) -> (-10.2329, 54.0174) construction
  line L113 (-10.8882, 53.5585) -> (-10.4294, 52.9032) construction
  line L114 (-10.5199, 55.6476) -> (-8.7991, 53.1902) construction
  line L115 (-8.7991, 53.1902) -> (-11.2566, 51.4694) construction
  line L116 (-11.2566, 51.4694) -> (-12.9773, 53.9269) construction
  line L117 (-12.9773, 53.9269) -> (-10.5199, 55.6476) construction
  line L118 (-10.5199, 55.6476) -> (-11.2566, 51.4694) construction
  line L119 (-8.7991, 53.1902) -> (-12.9773, 53.9269) construction
  circle A5 centre (-10.8882, 53.5585) radius 0.8 construction
  line L120 (-30.25, 11.5) -> (-30.25, 57) construction
  line L121 (30.25, 11.5) -> (30.25, 57) construction
  line L122 (-6.1403, 52) -> (6.1403, 52) construction
  line L123 (-31, 57) -> (-31, -30) construction
  line L124 (31, 57) -> (31, -30) construction
  line L125 (-30.25, 57) -> (-31, 57) construction
  line L126 (30.25, 57) -> (31, 57) construction
  line L127 (-31, 8.5) -> (31, 8.5) construction
  line L128 (-31, -8.5) -> (31, -8.5) construction
  circle A6 centre (0, 0) radius 7.5 construction
  line L129 (-31, -30) -> (31, -30) construction
  line L130 (-30.25, 44.8844) -> (-31, 44.3592) construction
  line L131 (-30.25, 35.1182) -> (-31, 34.593) construction
  line L132 (-26.25, 26.5) -> (-26.3613, 27.2922) construction
  line L133 (-26.25, 26.5) -> (-25.4578, 26.6113) construction
  line L134 (-29.0736, 28.6277) -> (-24.1223, 29.3236) construction
  line L135 (-24.1223, 29.3236) -> (-23.4264, 24.3723) construction
  line L136 (-23.4264, 24.3723) -> (-28.3777, 23.6764) construction
  line L137 (-28.3777, 23.6764) -> (-29.0736, 28.6277) construction
  line L138 (-29.0736, 28.6277) -> (-23.4264, 24.3723) construction
  line L139 (-24.1223, 29.3236) -> (-28.3777, 23.6764) construction
  circle A7 centre (-26.25, 26.5) radius 0.8 construction
  line L140 (-26.25, 57) -> (-26.25, -30) construction
  line L141 (-96, 180) -> (96, 180) construction
  line L142 (-26.3613, 27.2922) -> (-65.7556, 307.5968) construction
  line L143 (-186.6762, 186.6762) -> (-59.397, 313.9554) construction
  line L144 (59.397, 186.6762) -> (186.6762, 59.397) construction
  line L145 (-26.25, 26.5) -> (-80.4501, 292.9022) construction
  line L146 (-26.25, 26.5) -> (-47.9742, 302.5327) construction
  line L147 (63.6396, 190.9188) -> (-63.6396, 318.1981) construction
  line L148 (10.2335, 58.2897) -> (6.2185, 52.5556) projected
  line L149 (6.2185, 52.5556) -> (11.543, 48.8274) projected
  line L150 (11.543, 48.8274) -> (15.558, 54.5615) projected
  line L151 (15.558, 54.5615) -> (10.2335, 58.2897) construction
  line L152 (10.2335, 58.2897) -> (11.543, 48.8274) construction
  line L153 (6.2185, 52.5556) -> (15.558, 54.5615) construction
  line L154 (9.6599, 57.4705) -> (14.9844, 53.7423) construction
  line L155 (6.7921, 53.3748) -> (12.1165, 49.6465) construction
  line L156 (10.8882, 53.5585) -> (10.2329, 54.0174) construction
  line L157 (10.8882, 53.5585) -> (10.4294, 52.9032) construction
  line L158 (10.5199, 55.6476) -> (8.7991, 53.1902) construction
  line L159 (8.7991, 53.1902) -> (11.2566, 51.4694) construction
  line L160 (11.2566, 51.4694) -> (12.9773, 53.9269) construction
  line L161 (12.9773, 53.9269) -> (10.5199, 55.6476) construction
  line L162 (10.5199, 55.6476) -> (11.2566, 51.4694) construction
  line L163 (8.7991, 53.1902) -> (12.9773, 53.9269) construction
  circle A8 centre (10.8882, 53.5585) radius 0.8 construction
  line L164 (-24.1223, 29.3236) -> (-19.1709, 30.0195) construction
  line L165 (-19.1709, 30.0195) -> (-18.4751, 25.0681) construction
  line L166 (-18.4751, 25.0681) -> (-23.4264, 24.3723) construction
  line L167 (-24.1223, 29.3236) -> (-29.0736, 28.6277) construction
  line L168 (-29.0736, 28.6277) -> (-28.3777, 23.6764) construction
  line L169 (-28.3777, 23.6764) -> (-23.4264, 24.3723) construction
  line L170 (28.3777, 23.6764) -> (29.0736, 28.6277) construction
  line L171 (24.1223, 29.3236) -> (19.1709, 30.0195) construction
  line L172 (19.1709, 30.0195) -> (18.4751, 25.0681) construction
  line L173 (18.4751, 25.0681) -> (23.4264, 24.3723) construction
  line L174 (24.1223, 29.3236) -> (29.0736, 28.6277) construction
  line L175 (29.0736, 28.6277) -> (28.3777, 23.6764) construction
  line L176 (28.3777, 23.6764) -> (23.4264, 24.3723) construction
  line L177 (24.1223, 29.3236) -> (28.3777, 23.6764) construction
  line L178 (23.4264, 24.3723) -> (29.0736, 28.6277) construction
  line L179 (-21.2987, 27.1959) -> (-61.3286, 312.0238) construction
  line L180 (-21.2987, 27.1959) -> (-76.2182, 297.1342) construction
  line L181 (-21.2987, 27.1959) -> (-42.5405, 297.0989) construction
  line L182 (-24.1223, 29.3236) -> (-18.4751, 25.0681) construction
  line L183 (-23.4264, 24.3723) -> (-19.1709, 30.0195) construction
  line L184 (-15.558, 54.5615) -> (-18.0155, 52.8407) construction
  line L185 (-18.0155, 52.8407) -> (-14.0004, 47.1067) construction
  line L186 (-14.0004, 47.1067) -> (-11.543, 48.8274) construction
  point P0 (90, -90)
  point P1 (-90, -90)
  point P2 (-24.625, 0)
  point P3 (0, 61.1826)
  point P4 (-5.9733, 57)
  point P5 (-8.226, 55.4227)
  point P6 (0, 180)
  point P7 (8.226, 55.4227)
  constraints: 2 other
